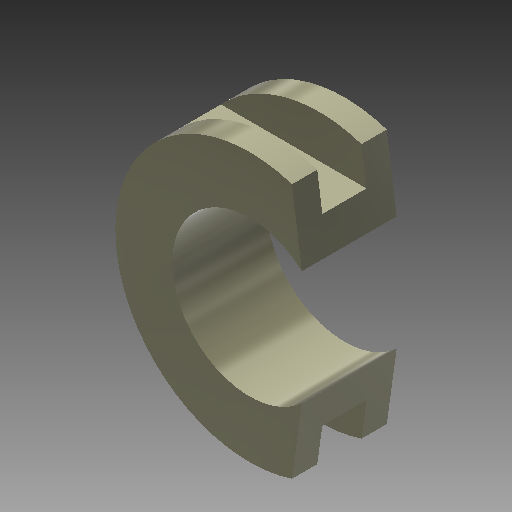
# Autodesk Inventor part: 308-03
Saved by Autodesk Inventor 2019 (Build 230136000, 136)
## iProperties
Company: Autodesk Inc.
Created: 2012-01-25
Part Number: 308-03
Material: Polypropylene
Document SubType Name: Modeling
Designer: Autodesk Inc.
Mass: 0.0543236 g
Surface Area: 1.59645 cm^2
Volume: 0.0604267 cm^3
Density: 0.899 g/cm^3
Appearance: Smooth - Ash
Author: Inventor
Autodesk Inventor part; units mm, degrees
ref_plane "YZ Plane" through (0, 0, 0) normal (1, 0, 0) x (0, 1, 0)
ref_plane "XZ Plane" through (0, 0, 0) normal (0, 1, 0) x (-1, 0, 0)
ref_plane "XY Plane" through (0, 0, 0) normal (0, 0, 1) x (1, 0, 0)
sketch "Sketch1" plane through (0, 0, 0) normal (0, 0, 1) x (1, 0, 0)
  circle A0 centre (0, 0) radius 4.25
  circle A1 centre (0, 0) radius 2.45
  line L0 (1.6512, 1.81) -> (1.3387, 4.0337)
  line L1 (1.3387, 4.0337) -> (1.3387, -4.0337) construction
  line L2 (1.3387, -4.0337) -> (1.6512, -1.81)
  line L3 (1.6512, 1.81) -> (1.6512, -1.81) construction
  dimension "d0" = 8.5
  dimension "d1" = 4.9
  dimension "d4" = 8
  dimension "d5" = 3.62
  constraints: 8 end point, 4 point on circle, 2 centre point, 2 coincident, 1 parallel, 1 vertical
  measures "d0" diameter of A0
  measures "d1" diameter of A1
  measures "d4" angle of L0 L1
  measures "d5" distance of L2.end L0.start
extrude "Extrusion1" add sketch "Sketch1" along normal mid plane 3 contours L0 A1 L2 A0 picked at (0.7697, -3.5469)
sketch "Sketch2" plane through (0, 0, 0) normal (1, 0, 0) x (0, 1, 0)
  line L0 (5.4492, 0.7) -> (2.9, 0.7)
  line L1 (2.9, 0.7) -> (2.9, -0.7)
  line L2 (2.9, -0.7) -> (5.7127, -0.7)
  line L3 (4.0337, 1.5) -> (1.81, 1.5) projected
  line L4 (1.81, -1.5) -> (4.0337, -1.5) projected
  point P0 (0, 0)
  dimension "d6" = 0.8
  dimension "d7" = 1.4
  dimension "d11" = 2.9
  constraints: 6 end point, 1 horizontal, 1 parallel, 1 perpendicular
  measures "d6" distance between parallel lines of L4 L2
  measures "d7" distance between parallel lines of L2 L0
  measures "d11" distance from line of point (0, 0) L1
extrude "Extrusion2" cut sketch "Sketch2" along normal through all both and the other way through all fills toward (4.1746, 0.65) open curves L0 L1 L2
mirror "Mirror1" about plane through (0, 0, 0) normal (0, 1, 0) of "Extrusion2"
body "Solid1"
